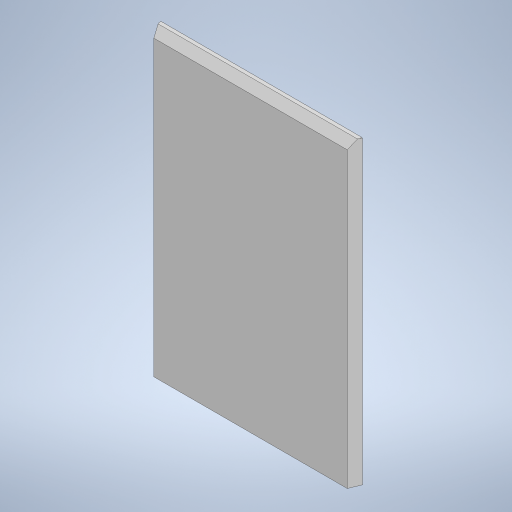
# Autodesk Inventor part: PotiBoxLid
Saved by Autodesk Inventor 2024.3 (Build 283343000, 343)
## iProperties
Created: 2025-03-30
Part Number: PotiBoxLid
Material: Generisch
Document SubType Name: Modeling
Designer: maxho
Density: 1 g/cm^3
Appearance: Vorgabe
Author: maxho
## iProperties of the stored document PotiBoxLid_3D-Druck.ipt
Created: 2025-03-30
Part Number: PotiBoxLid_3D-Druck
Material: Generisch
Document SubType Name: Modeling
Designer: maxho
Density: 1 g/cm^3
Appearance: Vorgabe
Author: maxho
Autodesk Inventor part; units mm, degrees
ref_plane "YZ Plane" through (0, 0, 0) normal (1, 0, 0) x (0, 1, 0)
ref_plane "XZ Plane" through (0, 0, 0) normal (0, 1, 0) x (-1, 0, 0)
ref_plane "XY Plane" through (0, 0, 0) normal (0, 0, 1) x (1, 0, 0)
sketch "Skizze1" plane through (0, 0, 0) normal (0, 0, 1) x (1, 0, 0)
  line L0 (0, 0) -> (-1.2426, 3)
  line L1 (-1.2426, 3) -> (54.6426, 3)
  line L2 (54.6426, 3) -> (53.4, 0)
  line L3 (53.4, 0) -> (0, 0)
  point P0 (26.7, 3)
  point P1 (26.7, 0)
  dimension "d1" = 112.5
  dimension "d2" = 3
  dimension "d3" = 53.4
  constraints: 8 end point, 2 midpoint, 1 horizontal, 1 parallel, 1 vertical alignment
  measures "d1" angle of L3 L0
  measures "d2" distance between parallel lines of L1 L3
  measures "d3" distance of L2.end L0.start
extrude "Extrusion1" add sketch "Skizze1" along normal blind 83
chamfer "Fasen1" distance 2 angle 45 1 edges at (26.7, 0, 83)
sketch "Skizze2" plane through (0, 0, 0) normal (0, -1, 0) x (1, 0, 0)
  line L0 (0, 81) -> (53.4, 81) projected
  line L1 (0, 0) -> (0, 81) projected
  line L2 (0, 0) -> (53.4, 0) projected
  line L3 (53.4, 0) -> (53.4, 81) projected
  line L4 (56.4, 81) -> (-3, 81)
  line L5 (-3, 81) -> (-1, 83)
  line L6 (-1, 83) -> (54.4, 83)
  line L7 (54.6426, 83) -> (-1.2426, 83) projected
  line L8 (54.4, 83) -> (56.4, 81)
  line L9 (0, 81) -> (53.4, 81) projected
  line L10 (-1.2426, 0) -> (-1.2426, 83) projected
  line L11 (54.6426, 0) -> (54.6426, 83) projected
  line L12 (-1, 83) -> (-1, 81)
  line L13 (54.4, 83) -> (54.4, 81)
  point P0 (26.7, 81)
  point P1 (26.7, 81)
  point P2 (26.7, 83)
  point P3 (-1.2426, 82.7574)
  point P4 (-1, 83)
  point P5 (54.6426, 82.7574)
  point P6 (55.4711, 85)
  point P7 (54.6426, 81)
  point P8 (-1.2426, 81)
  point P9 (-2.0711, 85)
  dimension "d9" = 59.4
  dimension "d10" = 45
  constraints: 12 end point, 5 midpoint, 2 point on line, 1 collinear, 1 horizontal, 1 perpendicular, 1 vertical, 1 vertical alignment
  measures "d9" distance of L4.start L4.end
  measures "d10" angle of L4 L8
extrude "Extrusion2" cut sketch "Skizze2" against normal through all contours L5 L10 L7 | L7 L11 L8
sketch "Skizze3" plane through (-1.2426, 3, 0) normal (0, 1, 0) x (1, 0, 0)
  line L0 (14.5597, -25.4927) -> (42.7158, -25.4927) construction
  line L1 (42.7158, -25.4927) -> (42.7158, -51.3659) construction
  line L2 (42.7158, -51.3659) -> (14.5597, -51.3659) construction
  line L3 (14.5597, -51.3659) -> (14.5597, -25.4927) construction
  line L4 (17.3308, -29.0636) -> (15.0192, -29.0636)
  line L5 (15.0192, -29.0636) -> (15.0192, -28.4538)
  line L6 (15.0192, -28.4538) -> (15.7566, -28.4538)
  line L7 (15.7566, -28.4538) -> (15.7566, -26.6017)
  line L8 (15.7566, -26.6017) -> (15.0192, -26.6017)
  line L9 (15.0192, -26.6017) -> (15.0192, -26.0316)
  spline S0 degree 2 poles (15.0192, -26.0316) (15.1809, -26.0316) (15.5014, -25.989) (15.5978, -25.9437) knots 0 0 0 1 2 2 2
  spline S1 degree 2 poles (15.5978, -25.9437) (15.7084, -25.8869) (15.8332, -25.6969) (15.8446, -25.5551) knots 0 0 0 1 2 2 2
  line L10 (15.8446, -25.5551) -> (16.6104, -25.5551)
  line L11 (16.6104, -25.5551) -> (16.6104, -28.4538)
  line L12 (16.6104, -28.4538) -> (17.3308, -28.4538)
  line L13 (17.3308, -28.4538) -> (17.3308, -29.0636)
  line L14 (18.7915, -29.0636) -> (17.9604, -29.0636)
  line L15 (17.9604, -29.0636) -> (17.9604, -28.139)
  line L16 (17.9604, -28.139) -> (18.7915, -28.139)
  line L17 (18.7915, -28.139) -> (18.7915, -29.0636)
  line L18 (21.9001, -29.0636) -> (19.5885, -29.0636)
  line L19 (19.5885, -29.0636) -> (19.5885, -28.4538)
  line L20 (19.5885, -28.4538) -> (20.3259, -28.4538)
  line L21 (20.3259, -28.4538) -> (20.3259, -26.6017)
  line L22 (20.3259, -26.6017) -> (19.5885, -26.6017)
  line L23 (19.5885, -26.6017) -> (19.5885, -26.0316)
  spline S2 degree 2 poles (19.5885, -26.0316) (19.7502, -26.0316) (20.0707, -25.989) (20.1671, -25.9437) knots 0 0 0 1 2 2 2
  spline S3 degree 2 poles (20.1671, -25.9437) (20.2777, -25.8869) (20.4025, -25.6969) (20.4139, -25.5551) knots 0 0 0 1 2 2 2
  line L24 (20.4139, -25.5551) -> (21.1797, -25.5551)
  line L25 (21.1797, -25.5551) -> (21.1797, -28.4538)
  line L26 (21.1797, -28.4538) -> (21.9001, -28.4538)
  line L27 (21.9001, -28.4538) -> (21.9001, -29.0636)
  line L28 (23.3608, -29.0636) -> (22.5297, -29.0636)
  line L29 (22.5297, -29.0636) -> (22.5297, -28.139)
  line L30 (22.5297, -28.139) -> (23.3608, -28.139)
  line L31 (23.3608, -28.139) -> (23.3608, -29.0636)
  spline S4 degree 2 poles (26.58, -27.3136) (26.58, -27.7674) (26.4353, -28.4481) (26.2737, -28.6779) knots 0 0 0 1 2 2 2
  spline S5 degree 2 poles (26.2737, -28.6779) (26.1148, -28.9048) (25.6015, -29.1373) (25.2327, -29.1373) knots 0 0 0 1 2 2 2
  spline S6 degree 2 poles (25.2327, -29.1373) (24.8612, -29.1373) (24.3506, -28.9048) (24.189, -28.6722) knots 0 0 0 1 2 2 2
  spline S7 degree 2 poles (24.189, -28.6722) (24.0273, -28.4424) (23.8827, -27.7674) (23.8827, -27.3136) knots 0 0 0 1 2 2 2
  spline S8 degree 2 poles (23.8827, -27.3136) (23.8827, -26.8484) (24.0273, -26.1904) (24.1918, -25.9522) knots 0 0 0 1 2 2 2
  spline S9 degree 2 poles (24.1918, -25.9522) (24.3563, -25.7196) (24.8754, -25.4927) (25.2327, -25.4927) knots 0 0 0 1 2 2 2
  spline S10 degree 2 poles (25.2327, -25.4927) (25.61, -25.4927) (26.1148, -25.7309) (26.2765, -25.9664) knots 0 0 0 1 2 2 2
  spline S11 degree 2 poles (26.2765, -25.9664) (26.4353, -26.1961) (26.58, -26.874) (26.58, -27.3136) knots 0 0 0 1 2 2 2
  spline S12 degree 2 poles (25.6979, -27.3136) (25.6979, -26.6641) (25.4852, -26.1394) (25.2327, -26.1394) knots 0 0 0 1 2 2 2
  spline S13 degree 2 poles (25.2327, -26.1394) (24.9803, -26.1394) (24.7647, -26.6641) (24.7647, -27.3164) knots 0 0 0 1 2 2 2
  spline S14 degree 2 poles (24.7647, -27.3164) (24.7647, -27.9574) (24.9803, -28.4907) (25.2327, -28.4907) knots 0 0 0 1 2 2 2
  spline S15 degree 2 poles (25.2327, -28.4907) (25.4823, -28.4907) (25.6979, -27.9574) (25.6979, -27.3136) knots 0 0 0 1 2 2 2
  point P0 (1.2426, 0)
  constraints: 2 other
emboss "Prägen1" sketch "Skizze3" operation cut depth 0.5 direction (0, -1, 0)
equation "\"d2\" = PotiBoxThickness"
equation "\"d3\" = PotiBoxInnerWidth"
equation "\"d4\" = PotiBoxInnerLength + PotiBoxThickness"
equation "\"d9\" = PotiBoxInnerWidth + 2 * PotiBoxThickness"
equation "\"PotiBoxThickness\" = 3"
equation "\"PotiBoxInnerWidth\" = 53.4"
equation "\"PotiBoxInnerLength\" = 80"
